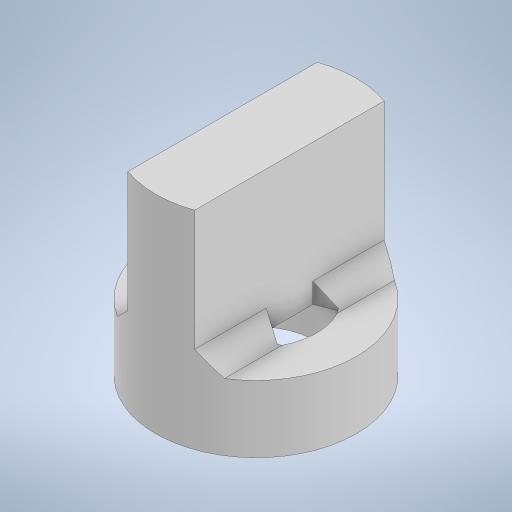
# Autodesk Inventor part: bone_attachment_3.0mm_test
Saved by Autodesk Inventor 2024 (Build 280153000, 153)
## iProperties
Created: 2024-06-07
Part Number: bone_attachment_3.0mm_test
Material: 일반
Document SubType Name: Modeling
Designer: Gihyeok Na
Density: 1 g/cm^3
Appearance: 기본값
Author: Gihyeok Na
Autodesk Inventor part; units mm, degrees
ref_plane "YZ Plane" through (0, 0, 0) normal (1, 0, 0) x (0, 1, 0)
ref_plane "XZ Plane" through (0, 0, 0) normal (0, 1, 0) x (-1, 0, 0)
ref_plane "XY Plane" through (0, 0, 0) normal (0, 0, 1) x (1, 0, 0)
sketch "스케치2" plane through (0, 0, 0) normal (0, 1, 0) x (-1, 0, 0)
  circle A0 centre (0, 0) radius 1.5
  circle A1 centre (0, 0) radius 0.9
  dimension "d0" = 3
  dimension "d6" = 1.8
  constraints: 2 centre point, 2 coincident
  measures "d0" diameter of A0
  measures "d6" diameter of A1
extrude "돌출1" add sketch "스케치2" along normal blind 1
sketch "스케치4" plane through (0, 1, 0) normal (0, 1, 0) x (1, 0, 0)
  line L0 (0.5, -1.55) -> (-0.5, -1.55)
  line L1 (-0.5, -1.55) -> (-0.5, 1.55)
  line L2 (-0.5, 1.55) -> (0.5, 1.55)
  line L3 (0.5, 1.55) -> (0.5, -1.55)
  line L4 (0.5, -1.55) -> (-0.5, 1.55) construction
  line L5 (-0.5, -1.55) -> (0.5, 1.55) construction
  circle A0 centre (0, 0) radius 1.5 projected
  point P0 (0.5, 1.4142)
  point P1 (-0.5, 1.4142)
  point P2 (-0.5, -1.4142)
  point P3 (0.5, -1.4142)
  dimension "d7" = 1
  constraints: 12 end point, 2 midpoint, 2 parallel, 1 horizontal, 1 perpendicular
  measures "d7" distance of L1.end L2.end
extrude "돌출3" add sketch "스케치4" along normal blind 2.1 contours A0 L1 L3
chamfer "모따기1" distance 0.3 angle 45 4 edges at (0.5, 1, 1.0813) (0.5, 1, -1.0813) (-0.5, 1, -1.0813) (-0.5, 1, 1.0813)
chamfer "모따기2" distance 0.4 angle 45 4 edges at (-0.5, 1.15, -0.7483) (-0.5, 1.15, 0.7483) (0.5, 1.15, 0.7483) (0.5, 1.15, -0.7483)
